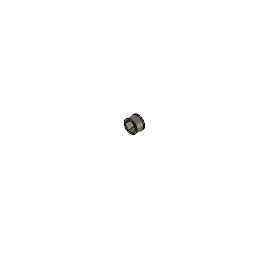
3-029 Hex Spacers (Autodesk Fusion 360 design; units mm, degrees)
Autodesk Fusion 360 part; units mm, degrees
ref_plane "WorkPlane1" through (0, 10, 0) normal (0, 1, 0) x (0, 0, 1)
sketch "Sketch1" plane through (0, 10, 0) normal (0, 1, 0) x (1, 0, 0)
  line L0 (-2.1, -3.6373) -> (2.1, -3.6373)
  line L1 (2.1, -3.6373) -> (4.2, 0)
  line L2 (4.2, 0) -> (2.1, 3.6373)
  line L3 (2.1, 3.6373) -> (-2.1, 3.6373)
  line L4 (-2.1, 3.6373) -> (-4.2, 0)
  line L5 (-4.2, 0) -> (-2.1, -3.6373)
  circle A0 centre (0, 0) radius 5
  dimension "d266" = 10
  dimension "d287" = 8.4
  constraint coincident A0.centre origin
  constraint horizontal L0
  measures "d266" diameter of A0
  measures "d287" distance of L0.start L2.end
extrude "Extrude1" add sketch "Sketch1" along normal blind 5 makes body 1
extrude "Extrude1'" add 1 faces at (-3.6016, 15, 1.9356) along direction (0, 1, 0) blind 1 separate body on bodies 1 makes body 2 in component "Component"
copy_body "Body->Comp1" bodies 1 removing the originals makes body 3 in component "Component'"
component "Component" placed x (1, 0, 0) y (0, 1, 0) z (0, 0, 1) at (0, 0, 0)
component "Component'" placed x (1, 0, 0) y (0, 1, 0) z (0, 0, 1) at (0, 0, 0)
